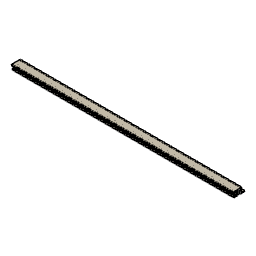
tip top audio zrail profile (Autodesk Fusion 360 design; units mm, degrees)
Autodesk Fusion 360 part; units mm, degrees
sketch "Sketch1" plane through (0, 0, 0) normal (1, 0, 0) x (0, 0, -1)
  line L0 (-14.3, 5) -> (3.5, 5)
  line L1 (3.5, 5) -> (3.5, 3.8)
  line L2 (3.5, 3.8) -> (1.5, 3.8)
  line L3 (1.5, 3.8) -> (1.5, 2.4)
  line L4 (1.5, 2.4) -> (3.5, 2.4)
  line L5 (3.5, 2.4) -> (3.5, 0.6521)
  line L6 (3.5, 0.6521) -> (1.5157, 0.6521)
  line L7 (-14.3, 5) -> (-14.3, 3.8)
  line L8 (-14.3, 3.8) -> (-11.5, 3.8)
  line L9 (-11.5, 3.8) -> (-11.5, 2)
  line L10 (-11.5, 2) -> (-9.4055, 2)
  line L11 (-9.4055, 2) -> (-9.4055, 3.25)
  line L12 (-9.4055, 3.25) -> (-6.9619, 3.25)
  line L13 (-6.9619, 3.25) -> (-6.9619, 2)
  line L14 (-6.9619, 2) -> (-3.9, 2)
  line L15 (-3.9, 2) -> (-3.9, -2)
  line L16 (-3.9, -2) -> (-6.9619, -2)
  line L17 (-6.9619, -2) -> (-6.9619, -3.25)
  line L18 (-6.9619, -3.25) -> (-9.4055, -3.25)
  line L19 (-9.4055, -3.25) -> (-9.4055, -2)
  line L20 (-9.4055, -2) -> (-11.5, -2)
  line L21 (-11.5, -2) -> (-11.5, -5)
  line L22 (-11.5, -5) -> (-5, -5)
  line L23 (-5, -5) -> (-5, -3.8)
  line L24 (-5, -3.8) -> (0, -3.8)
  line L25 (0, -3.8) -> (0, -5)
  line L26 (0, -5) -> (9.5, -5)
  line L27 (9.5, -5) -> (9.5, -3.8)
  line L28 (9.5, -3.8) -> (3.5, -3.8)
  line L29 (3.5, -3.8) -> (3.5, -0.3575)
  line L30 (3.5, -0.3575) -> (1.6108, -0.3575)
  arc A0 (1.5157, 0.6521) -> (1.6108, -0.3575) centre (0, 0) ccw
  dimension "d1" = 5
  dimension "d2" = 6.5
  dimension "d3" = 4
  dimension "d4" = 3
  dimension "d5" = 1.2
  dimension "d6" = 10
  dimension "d7" = 2.8
  dimension "d8" = 7.6
  dimension "d9" = 1.4
  dimension "d10" = 1.2
  dimension "d11" = 6
  dimension "d12" = 9.5
  dimension "d13" = 2
  dimension "d14" = 23.8
  dimension "d15" = 1.2
  dimension "d16" = 1.65
  dimension "d17" = 3.5
  dimension "d18" = 3.8
  dimension "d19" = 5
  dimension "d20" = 1.75
  constraint horizontal L0
  constraint perpendicular L0 L1
  constraint perpendicular L1 L2
  constraint perpendicular L0 L3
  constraint perpendicular L1 L4
  constraint perpendicular L2 L5
  constraint perpendicular L5 L6
  constraint perpendicular L0 L7
  constraint perpendicular L7 L8
  constraint perpendicular L8 L9
  constraint perpendicular L9 L10
  constraint perpendicular L10 L11
  constraint perpendicular L9 L12
  constraint perpendicular L12 L13
  constraint perpendicular L13 L14
  constraint perpendicular L14 L15
  constraint perpendicular L15 L16
  constraint perpendicular L14 L17
  constraint perpendicular L15 L18
  constraint perpendicular L18 L19
  constraint perpendicular L19 L20
  constraint perpendicular L20 L21
  constraint perpendicular L21 L22
  constraint perpendicular L22 L23
  constraint perpendicular L23 L24
  constraint perpendicular L24 L25
  constraint perpendicular L23 L26
  constraint perpendicular L26 L27
  constraint perpendicular L27 L28
  constraint perpendicular L28 L29
  constraint perpendicular L29 L30
  constraint collinear L1 L5
  constraint collinear L5 L29
  constraint collinear L10 L14
  constraint collinear L16 L20
  constraint collinear L13 L17
  constraint collinear L11 L19
  constraint collinear L9 L21
  constraint coincident A0.centre origin
  constraint collinear L22 L26
  measures "d1" distance of L23.end L24.end
  measures "d2" distance of L12 L18
  measures "d3" distance of L10 L20
  measures "d4" distance of L20 L22
  measures "d5" distance of L0.start L7.end
  measures "d6" distance of L0 L22
  measures "d7" distance of L7.end L8.end
  measures "d8" distance of L9 L15
  measures "d9" distance of L2 L4
  measures "d10" distance of L0.end L1.end
  measures "d11" distance of L27 L29
  measures "d12" distance of L25 L27
  measures "d13" distance of L1.end L2.end
  measures "d14" distance of L7 L27
  measures "d15" distance of L22 L24
  measures "d16" radius of A0
  measures "d17" distance of L1 A0.centre
  measures "d18" distance of L28 A0.centre
  measures "d19" distance of L0 A0.centre
  measures "d20" distance of L0 L12
extrude "Extrude1" add sketch "Sketch1" along normal blind 426.72
equation "d16 = ( 3.3 / 2 ) * 1 mm"
equation "d20 = ( d6 - d2 ) / 2"
equation "d21 = hp_constant * hp_units"
equation "hp_units = 84"
equation "hp_constant = 5.08 mm"
